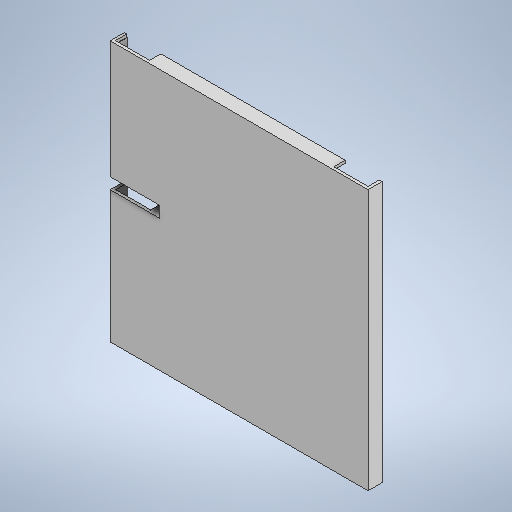
# Autodesk Inventor part: 2025_03_10_Reaktor_oben
Saved by Autodesk Inventor 2025.1 (Build 291241000, 241)
## iProperties
Created: 2020-10-19
Part Number: 2025_03_10_Reaktor_oben
Material: ABS-Kunststoff
Document SubType Name: Modeling
Designer: Daniel
Density: 1.06 g/cm^3
Appearance: Vorgabe
Author: Daniel
Autodesk Inventor part; units mm, degrees
ref_plane "YZ Plane" through (0, 0, 0) normal (1, 0, 0) x (0, 1, 0)
ref_plane "XZ Plane" through (0, 0, 0) normal (0, 1, 0) x (-1, 0, 0)
ref_plane "XY Plane" through (0, 0, 0) normal (0, 0, 1) x (1, 0, 0)
sketch "Skizze1" plane through (0, 0, 0) normal (0, 0, 1) x (1, 0, 0)
  line L0 (-64.7, -64.7) -> (64.7, -64.7)
  line L1 (64.7, -64.7) -> (64.7, 64.7)
  line L2 (64.7, 64.7) -> (-64.7, 64.7)
  line L3 (-64.7, 64.7) -> (-64.7, -64.7)
  line L4 (-64.7, -64.7) -> (64.7, 64.7) construction
  line L5 (64.7, -64.7) -> (-64.7, 64.7) construction
  point P0 (0, 0)
  dimension "d0" = 129.4
  dimension "d1" = 129.4
  constraints: 12 end point, 2 midpoint, 2 parallel, 1 horizontal, 1 perpendicular
  measures "d0" distance of L1.end L2.end
  measures "d1" distance of L0.end L1.end
extrude "Extrusion1" add sketch "Skizze1" along normal blind 22
sketch "Skizze2" plane through (0, 0, 22) normal (0, 0, 1) x (1, 0, 0)
  line L0 (-132.05, 89.45) -> (128.95, 89.45)
  line L1 (64.7, 64.7) -> (-64.7, 64.7) projected
  line L2 (89.45, 116.05) -> (89.45, -84.95)
  line L3 (-89.45, 121.95) -> (-89.45, -89.05)
  line L4 (64.7, -64.7) -> (64.7, 64.7) projected
  line L5 (-64.7, 64.7) -> (-64.7, -64.7) projected
  line L6 (-157.95, -91.45) -> (148.05, -91.45)
  line L7 (-64.7, -64.7) -> (64.7, -64.7) projected
  line L8 (89.45, -84.95) -> (89.45, -91.95)
  line L9 (-89.45, -89.05) -> (-89.45, -94.05)
  point P0 (0, 0)
  point P1 (-89.45, -91.45)
  point P2 (89.45, -91.45)
  point P3 (89.45, 89.45)
  point P4 (-89.45, 89.45)
  dimension "d4" = 24.75
  dimension "d5" = 24.75
  dimension "d6" = 24.75
  dimension "d7" = 26.75
  constraints: 12 end point, 2 horizontal, 2 perpendicular, 2 vertical
  measures "d4" distance between parallel lines of L1 L0
  measures "d5" distance between parallel lines of L4 L2
  measures "d6" distance between parallel lines of L5 L3
  measures "d7" distance between parallel lines of L6 L7
extrude "Extrusion2" add sketch "Skizze2" along normal blind 2 contours L0 L2 L8 L6 L9 L3 | L4 L7 L5 L1
sketch "Skizze3" plane through (0, 0, 24) normal (0, 0, 1) x (1, 0, 0)
  line L0 (-91.45, 91.45) -> (91.45, 91.45)
  line L1 (91.45, 91.45) -> (91.45, -93.45)
  line L2 (91.45, -93.45) -> (-91.45, -93.45)
  line L3 (-91.45, -93.45) -> (-91.45, 91.45)
  line L4 (89.45, 89.45) -> (-89.45, 89.45) projected
  line L5 (-89.45, 89.45) -> (-89.45, -91.45) projected
  line L6 (89.45, -91.45) -> (89.45, 89.45) projected
  line L7 (-89.45, -91.45) -> (89.45, -91.45) projected
  line L8 (-89.45, 89.45) -> (-89.45, -91.45) projected
  line L9 (-89.45, 89.45) -> (89.45, 89.45)
  line L10 (89.45, 89.45) -> (89.45, -91.45)
  line L11 (89.45, -91.45) -> (-89.45, -91.45)
  line L12 (-89.45, -91.45) -> (-89.45, 89.45)
  point P0 (0, 0)
  dimension "d10" = 2
  dimension "d11" = 2
  dimension "d12" = 2
  dimension "d13" = 2
  constraints: 16 end point, 4 parallel, 2 horizontal, 2 perpendicular
  measures "d10" distance between parallel lines of L4 L0
  measures "d11" distance between parallel lines of L5 L3
  measures "d12" distance between parallel lines of L6 L1
  measures "d13" distance between parallel lines of L2 L7
extrude "Extrusion3" add sketch "Skizze3" against normal blind 10
sketch "Skizze4" plane through (0, 0, 14) normal (0, 0, -1) x (-1, 0, 0)
  line L0 (89.45, -91.45) -> (-89.45, -91.45) projected
  line L1 (-91.45, -93.45) -> (91.45, -93.45) projected
  line L2 (89.45, -91.45) -> (64.95, -91.45)
  line L3 (64.95, -91.45) -> (64.95, -93.45)
  line L4 (64.95, -93.45) -> (89.45, -93.45)
  line L5 (89.45, -93.45) -> (89.45, -91.45)
  line L6 (-89.45, -91.45) -> (-64.95, -91.45)
  line L7 (-64.95, -91.45) -> (-64.95, -93.45)
  line L8 (-64.95, -93.45) -> (-89.45, -93.45)
  line L9 (-89.45, -93.45) -> (-89.45, -91.45)
  point P0 (0, 0)
  point P1 (89.45, -93.45)
  point P2 (-89.45, -91.45)
  point P3 (-89.45, -93.45)
  point P4 (-64.95, -93.45)
  point P5 (-64.95, -91.45)
  dimension "d16" = 24.5
  dimension "d17" = 24.5
  constraints: 16 end point, 4 parallel, 3 point on line, 2 horizontal, 2 perpendicular
  measures "d16" distance between parallel lines of L9 L7
  measures "d17" distance between parallel lines of L5 L3
extrude "Extrusion4" cut sketch "Skizze4" against normal up to surface (8 mm away) contours L5 L1 L3 L0 | L7 L1 L9 L0
sketch "Skizze6" plane through (91.45, -93.45, 24) normal (1, 0, 0) x (0, 0, -1)
  line L0 (10, 0) -> (10, 182.9) projected
  line L1 (0, 0) -> (10, 0)
  line L2 (10, 0) -> (10, 27)
  line L3 (10, 27) -> (0, 27)
  line L4 (0, 27) -> (0, 0)
  line L5 (0, 184.9) -> (10, 184.9) projected
  line L6 (0, 184.9) -> (10, 184.9)
  line L7 (10, 184.9) -> (10, 157.9)
  line L8 (10, 157.9) -> (0, 157.9)
  line L9 (0, 157.9) -> (0, 184.9)
  point P0 (24, 93.45)
  dimension "d20" = 27
  dimension "d21" = 27
  constraints: 16 end point, 4 parallel, 2 horizontal, 2 perpendicular, 2 point on line
  measures "d20" distance of L3.end L1.start
  measures "d21" distance of L8.end L5.start
extrude "Extrusion5" cut sketch "Skizze6" against normal up to surface (2 mm away)
sketch "Skizze7" plane through (-91.45, 91.45, 24) normal (0, 1, 0) x (1, 0, 0)
  line L0 (182.9, 10) -> (180.9, 10) projected
  line L1 (180.9, 10) -> (180.9, 2) projected
  line L2 (180.9, 0) -> (0, 0) projected
  line L3 (182.9, 10) -> (182.9, 0) projected
  line L4 (181.15, 2) -> (156.65, 2)
  line L5 (156.65, 2) -> (156.65, 10)
  line L6 (156.65, 10) -> (181.15, 10)
  line L7 (181.15, 10) -> (181.15, 2)
  line L8 (180.9, 10) -> (2, 10) projected
  line L9 (0, 0) -> (0, 10) projected
  line L10 (1.75, 2) -> (26, 2)
  line L11 (26, 2) -> (26, 10)
  line L12 (26, 10) -> (1.75, 10)
  line L13 (1.75, 10) -> (1.75, 2)
  point P0 (91.45, 24)
  point P1 (181.15, 10)
  point P2 (1.75, 10)
  point P3 (2, 10)
  point P4 (180.9, 10)
  dimension "d26" = 1.75
  dimension "d27" = 24.25
  dimension "d28" = 1.75
  dimension "d29" = 2
  dimension "d30" = 1.75
  dimension "d31" = 2
  dimension "d32" = 1.75
  dimension "d33" = 24.25
  constraints: 16 end point, 4 parallel, 3 point on line, 2 horizontal, 2 perpendicular
  measures "d26" distance from line of L3 point (181.15, 10)
  measures "d27" distance of L5.end L0.end
  measures "d28" distance from line of L3 L4.start
  measures "d29" vertical distance of L2.start L4.start
  measures "d30" distance from line of L9 point (1.75, 10)
  measures "d31" distance from line of L2 L10.start
  measures "d32" distance from line of L9 L10.start
  measures "d33" distance of L11.end point (1.75, 10)
extrude "Extrusion6" cut sketch "Skizze7" against normal blind 2 contours L11 L10 L13 L12 L8 | L1 L4 L5 L6
sketch "Skizze8" plane through (91.45, -66.45, 24) normal (1, 0, 0) x (0, 0, -1)
  line L0 (10, -27) -> (2, -27) projected
  line L1 (0, 157.9) -> (10, 157.9) projected
  line L2 (10, -27) -> (0, -27)
  line L3 (0, -27) -> (0, 157.9)
  line L4 (0, 157.9) -> (10, 157.9)
  line L5 (10, 157.9) -> (10, -27)
  point P0 (24, 66.45)
  constraints: 8 end point, 2 parallel, 1 horizontal, 1 perpendicular
extrude "Extrusion7" add sketch "Skizze8" against normal blind 2
sketch "Skizze18" plane through (-91.45, -93.45, 24) normal (-1, 0, 0) x (0, 0, 1)
  line L0 (-24, 93.45) -> (0, 93.45)
  line L1 (0, 93.45) -> (0, 101.45)
  line L2 (0, 101.45) -> (-24, 101.45)
  line L3 (-24, 101.45) -> (-24, 93.45)
  dimension "d97" = 24
  dimension "d98" = 8
  constraints: 8 end point, 2 parallel, 1 horizontal, 1 perpendicular
  measures "d97" distance of L2.end L1.end
  measures "d98" distance of L1.end L0.end
extrude "Extrusion17" cut sketch "Skizze18" against normal blind 35
